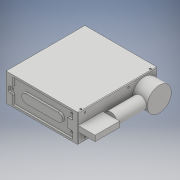
# Autodesk Inventor part: Syringe Pump
Saved by Autodesk Inventor 2018.1 (Build 221171000, 171)
## iProperties
Created: 2024-05-29
Part Number: Syringe Pump
Material: Generic
Document SubType Name: Modeling
Designer: em2714
Density: 1 g/cm^3
Appearance: Default
Author: em2714
Autodesk Inventor part; units mm, degrees
ref_plane "YZ Plane" through (0, 0, 0) normal (1, 0, 0) x (0, 1, 0)
ref_plane "XZ Plane" through (0, 0, 0) normal (0, 1, 0) x (-1, 0, 0)
ref_plane "XY Plane" through (0, 0, 0) normal (0, 0, 1) x (1, 0, 0)
sketch "Sketch1" plane through (0, 0, 0) normal (0, 1, 0) x (-1, 0, 0)
  line L0 (58.1, 22.5) -> (-58.1, 22.5)
  line L1 (-58.1, 22.5) -> (-58.1, -22.5)
  line L2 (-58.1, -22.5) -> (58.1, -22.5)
  line L3 (58.1, -22.5) -> (58.1, 22.5)
  point P0 (0, 0)
  point P1 (-58.1, 0)
  point P2 (0, -22.5)
  dimension "d0" = 116.2
  dimension "d1" = 45
  constraints: 8 end point, 2 midpoint, 2 parallel, 1 horizontal, 1 horizontal alignment, 1 perpendicular, 1 vertical alignment
  measures "d0" distance of L1.end L2.end
  measures "d1" distance between parallel lines of L2 L0
extrude "Extrusion1" add sketch "Sketch1" along normal mid plane 127
sketch "Sketch2" plane through (-58.1, 63.5, 22.5) normal (0, 0, 1) x (1, 0, 0)
  circle A0 centre (113.2, -120) radius 1.5
  circle A1 centre (113.2, -8) radius 1.5
  line L0 (116.2, -127) -> (0, -127) projected
  line L1 (116.2, -127) -> (116.2, 0) projected
  point P0 (58.1, -63.5)
  dimension "d6" = 3
  dimension "d8" = 3
  dimension "d9" = 7
  dimension "d10" = 112
  dimension "d11" = 3
  constraints: 2 centre point, 1 vertical alignment
  measures "d6" diameter of A0
  measures "d8" distance from line of L1 A0.centre
  measures "d9" distance from line of L0 A0.centre
  measures "d10" distance of A0.centre A1.centre
  measures "d11" diameter of A1
extrude "Extrusion2" cut sketch "Sketch2" against normal blind 1
mirror "Mirror1" about plane through (0, 0, 0) normal (0, 0, 1) of "Extrusion2"
sketch "Sketch3" plane through (58.1, -63.5, -22.5) normal (1, 0, 0) x (0, 0, -1)
  circle A0 centre (-39.75, 11) radius 1.5
  line L0 (0, 0) -> (-45, 0) construction
  line L1 (-45, 0) -> (-45, 127) construction
  circle A1 centre (-39.75, 81) radius 1.5
  line L2 (-22.5, 63.5) -> (-22.5, 0) construction
  circle A2 centre (-5.25, 11) radius 1.5
  circle A3 centre (-5.25, 81) radius 1.5
  dimension "d14" = 3
  dimension "d15" = 11
  dimension "d17" = 3
  dimension "d18" = 70
  dimension "d65" = 34.5
  constraints: 4 centre point, 2 end point, 2 symmetric about line, 1 midpoint, 1 vertical alignment, 2 other
  measures "d14" diameter of A0
  measures "d15" distance from line of L0 A0.centre
  measures "d17" diameter of A1
  measures "d18" distance of A0.centre A1.centre
  measures "d65" distance of A3.centre A1.centre
extrude "Extrusion3" cut sketch "Sketch3" against normal blind 1
sketch "Sketch4" plane through (0, 63.5, 0) normal (0, 1, 0) x (1, 0, 0)
  circle A0 centre (55.1, 16.5) radius 1.5
  line L0 (58.1, -22.5) -> (58.1, 22.5) construction
  line L1 (58.1, 22.5) -> (-58.1, 22.5) construction
  circle A1 centre (55.1, -16.5) radius 1.5
  line L2 (-58.1, -22.5) -> (58.1, -22.5) projected
  line L3 (0, 0) -> (58.1, 0)
  line L4 (58.1, 22.5) -> (58.1, -22.5) projected
  dimension "d21" = 3
  dimension "d22" = 3
  dimension "d24" = 3
  dimension "d25" = 33
  constraints: 2 centre point, 2 end point, 1 midpoint, 1 symmetric about line, 1 vertical alignment
  measures "d21" diameter of A0
  measures "d22" distance from line of L0 A0.centre
  measures "d24" diameter of A1
  measures "d25" distance of A0.centre A1.centre
extrude "Extrusion4" cut sketch "Sketch4" against normal blind 1
chamfer "Chamfer1" distance 1 angle 45 4 edges at (58.1, 63.5, 0) (58.1, 0, 22.5) (58.1, 0, -22.5) (58.1, -63.5, 0)
sketch "Sketch5" plane through (0, -63.5, 0) normal (0, -1, 0) x (1, 0, 0)
  line L0 (40.1, 5.5) -> (40.1, -5.5)
  line L1 (47.6, -19.5) -> (-47.1, -19.5)
  line L2 (-47.1, -19.5) -> (-47.1, -6.5)
  line L3 (-49.1, -4.5) -> (-52.1, -4.5)
  line L4 (-54.1, -2.5) -> (-54.1, 2.5)
  line L5 (-52.1, 4.5) -> (-49.1, 4.5)
  line L6 (-47.1, 6.5) -> (-47.1, 19.5)
  line L7 (-47.1, 19.5) -> (47.6, 19.5)
  line L8 (57.1, 22.5) -> (57.1, -22.5) construction
  line L9 (57.1, 0) -> (-58.1, 0) construction
  line L10 (-58.1, 22.5) -> (-58.1, -22.5) construction
  line L11 (42.1, -7.5) -> (47.6, -7.5)
  line L12 (49.6, -9.5) -> (49.6, -17.5)
  line L13 (42.1, 7.5) -> (47.6, 7.5)
  line L14 (49.6, 9.5) -> (49.6, 17.5)
  line L15 (-58.1, -22.5) -> (57.1, -22.5) projected
  arc A0 (-49.1, 4.5) -> (-47.1, 6.5) centre (-49.1, 6.5) ccw
  arc A1 (-47.1, -6.5) -> (-49.1, -4.5) centre (-49.1, -6.5) ccw
  arc A2 (-52.1, 4.5) -> (-54.1, 2.5) centre (-52.1, 2.5) ccw
  arc A3 (-54.1, -2.5) -> (-52.1, -4.5) centre (-52.1, -2.5) ccw
  arc A4 (42.1, 7.5) -> (40.1, 5.5) centre (42.1, 5.5) ccw
  arc A5 (47.6, 7.5) -> (49.6, 9.5) centre (47.6, 9.5) ccw
  arc A6 (49.6, -9.5) -> (47.6, -7.5) centre (47.6, -9.5) ccw
  arc A7 (47.6, -19.5) -> (49.6, -17.5) centre (47.6, -17.5) ccw
  arc A8 (49.6, 17.5) -> (47.6, 19.5) centre (47.6, 17.5) ccw
  arc A9 (40.1, -5.5) -> (42.1, -7.5) centre (42.1, -5.5) ccw
  circle A10 centre (-49.9, 0) radius 1.5
  circle A11 centre (44.1, 13) radius 1.5
  line L16 (57.1, 22.5) -> (-58.1, 22.5) projected
  circle A12 centre (44.1, -13) radius 1.5
  point P0 (0, 0)
  point P1 (-47.1, 4.5)
  point P2 (49.6, 7.5)
  dimension "d32" = 17
  dimension "d33" = 4
  dimension "d34" = 11
  dimension "d35" = 9
  dimension "d36" = 3
  dimension "d37" = 2
  dimension "d38" = 15
  dimension "d39" = 7.5
  dimension "d40" = 2
  dimension "d41" = 3
  dimension "d42" = 8.2
  dimension "d43" = 3
  dimension "d44" = 9.5
  dimension "d45" = 13
  dimension "d68" = 22.5
  constraints: 26 end point, 20 point on circle, 20 tangent, 13 centre point, 8 equal radius, 8 perpendicular, 8 point on line, 2 midpoint, 1 horizontal, 1 symmetric about line, 1 vertical, 5 other
  measures "d32" distance between parallel lines of L0 L8
  measures "d33" distance between parallel lines of L10 L4
  measures "d34" distance between parallel lines of L10 L2
  measures "d35" distance between parallel lines of L3 L5
  measures "d36" distance between parallel lines of L15 L1
  measures "d37" radius of A0
  measures "d38" distance between parallel lines of L11 L13
  measures "d39" distance between parallel lines of L8 L12
  measures "d40" radius of A4
  measures "d41" diameter of A10
  measures "d42" distance of L9.end A10.centre
  measures "d43" diameter of A11
  measures "d44" distance from line of A11.centre L16
  measures "d45" distance from line of L8 A11.centre
  measures "d68" distance from line of L15 A10.centre
extrude "Extrusion5" cut sketch "Sketch5" against normal blind 3
sketch "Sketch6" plane through (0, -63.5, 0) normal (0, -1, 0) x (1, 0, 0)
  circle A0 centre (44.1, 13) radius 1.5 projected
  circle A1 centre (44.1, -13) radius 1.5 projected
  circle A2 centre (-49.9, 0) radius 1.5 projected
  point P0 (0, 0)
extrude "Extrusion6" cut sketch "Sketch6" against normal blind 4
sketch "Sketch7" plane through (0, -60.5, 0) normal (0, -1, 0) x (1, 0, 0)
  line L0 (-26, 0) -> (26, 0) construction
  line L1 (-26, 7) -> (26, 7)
  line L2 (26, -7) -> (-26, -7)
  arc A0 (-26, 7) -> (-26, -7) centre (-26, 0) ccw
  arc A1 (26, -7) -> (26, 7) centre (26, 0) ccw
  point P0 (0, 0)
  dimension "d50" = 14
  dimension "d51" = 52
  constraints: 8 end point, 4 point on circle, 4 tangent, 2 centre point, 1 horizontal, 1 midpoint, 1 parallel
  measures "d50" distance between parallel lines of L2 L1
  measures "d51" distance of L0.start L0.end
extrude "Extrusion7" add sketch "Sketch7" along normal up to surface (3 mm away)
sketch "Sketch8" plane through (58.1, -62.5, 21.5) normal (1, 0, 0) x (0, 0, -1)
  circle A0 centre (21.5, 105.5) radius 19.5
  line L0 (44, 126) -> (-1, 126) projected
  point P0 (21.5, 62.5)
  dimension "d54" = 39
  dimension "d55" = 20.5
  constraints: 1 centre point, 1 vertical alignment
  measures "d54" diameter of A0
  measures "d55" distance from line of L0 A0.centre
extrude "Extrusion8" add sketch "Sketch8" along normal blind 24
ref_plane "Work Plane1" through (58.1, 23.5, 0) normal (0, 1, 0) x (-1, 0, 0)
sketch "Sketch9" plane through (58.1, 23.5, 0) normal (0, 1, 0) x (-1, 0, 0)
  line L0 (-24, 19.5) -> (-24, -19.5) projected
  circle A0 centre (-13, 0) radius 10
  point P0 (58.1, 0)
  point P1 (-24, 0)
  point P2 (-23, 0)
  dimension "d58" = 20
  dimension "d59" = 1
  constraints: 3 horizontal alignment, 1 midpoint, 2 other
  measures "d59" distance of point (-24, 0) point (-23, 0)
extrude "Extrusion9" add sketch "Sketch9" against normal blind 47.5
sketch "Sketch10" plane through (71.1, -24, 0) normal (0, -1, 0) x (1, 0, 0)
  line L0 (-13, -21.5) -> (-13, 21.5) projected
  line L1 (14.1, 4.5) -> (-13, 4.5)
  line L2 (-13, 4.5) -> (-13, -4.5)
  line L3 (-13, -4.5) -> (14.1, -4.5)
  line L4 (14.1, -4.5) -> (14.1, 4.5)
  line L5 (14.1, 0) -> (-13, 0) construction
  line L6 (11, -19.5) -> (11, 19.5) projected
  point P0 (-71.1, 0)
  point P1 (11, 0)
  dimension "d62" = 9
  dimension "d66" = 27.1
  dimension "d67" = 24
  constraints: 10 end point, 3 midpoint, 2 parallel, 2 perpendicular, 2 point on line, 1 horizontal, 1 other
  measures "d62" distance between parallel lines of L3 L1
  measures "d66" distance of L2.end L3.end
  measures "d67" distance between parallel lines of L0 L6
extrude "Extrusion10" add sketch "Sketch10" along normal up to surface (39.5 mm away)
body "Solid1"
